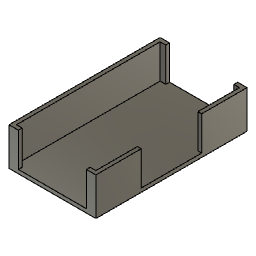
amp box v1 (Autodesk Fusion 360 design; units mm, degrees)
Autodesk Fusion 360 part; units mm, degrees
sketch "Sketch1" plane through (0, 0, 0) normal (0, 0, 1) x (1, 0, 0)
  line L0 (0, 0) -> (46, 0)
  line L1 (46, 0) -> (46, 80)
  line L2 (46, 80) -> (0, 80)
  line L3 (0, 80) -> (0, 0)
  dimension "d1" = 46
  dimension "d2" = 80
  constraint horizontal L0
  constraint vertical L1
  constraint horizontal L2
  constraint vertical L3
  constraint coincident L0.start L3.end
  measures "d1" distance of L0.start L0.end
  measures "d2" distance of L0.start L2.end
extrude "Extrude1" add sketch "Sketch1" along normal blind 20
shell "Shell1" thickness 2 removed faces 1 at (15.3333, 53.3333, 20)
sketch "Sketch2" plane through (0, 0, 0) normal (0, -1, 0) x (1, 0, 0)
  line L0 (0, 0) -> (46, 0)
  line L1 (46, 0) -> (46, 20)
  line L2 (46, 20) -> (0, 20)
  line L3 (0, 20) -> (0, 0)
  line L4 (46, 20) -> (41, 20)
  line L5 (41, 20) -> (41, -16.068)
  line L6 (41, -16.068) -> (46, -16.068)
  line L7 (46, -16.068) -> (46, 20)
  line L8 (0, 0) -> (5, 0)
  line L9 (5, 0) -> (5, 36.068)
  line L10 (5, 36.068) -> (0, 36.068)
  line L11 (0, 36.068) -> (0, 0)
  line L12 (46, 0) -> (0, 0)
  line L13 (0, 0) -> (0, 2)
  line L14 (0, 2) -> (46, 2)
  line L15 (46, 2) -> (46, 0)
  dimension "d6" = 5
  dimension "d7" = 5
  dimension "d8" = 2
  constraint horizontal L4
  constraint vertical L5
  constraint horizontal L6
  constraint vertical L7
  constraint coincident L1.end L2.start
  constraint horizontal L8
  constraint vertical L9
  constraint horizontal L10
  constraint vertical L11
  constraint coincident L0.start L3.end
  constraint horizontal L12
  constraint vertical L13
  constraint horizontal L14
  constraint vertical L15
  constraint coincident L0.end L1.start
  measures "d6" distance of L1.end L4.end
  measures "d7" distance of L0.start L8.end
  measures "d8" distance of L0.end L14.end
extrude "Extrude2" cut sketch "Sketch2" against normal blind 155 contours L2 L5 L9 L14
sketch "Sketch3" plane through (46, 0, 0) normal (1, 0, 0) x (0, 1, 0)
  line L0 (0, 0) -> (80, 0)
  line L1 (80, 0) -> (80, 20)
  line L2 (80, 20) -> (0, 20)
  line L3 (0, 20) -> (0, 0)
  line L4 (80, 0) -> (56, 0)
  line L5 (56, 0) -> (56, 36.068)
  line L6 (56, 36.068) -> (80, 36.068)
  line L7 (80, 36.068) -> (80, 0)
  line L8 (0, 20) -> (24, 20)
  line L9 (24, 20) -> (24, -16.068)
  line L10 (24, -16.068) -> (0, -16.068)
  line L11 (0, -16.068) -> (0, 20)
  line L12 (0, 0) -> (142, 0)
  line L13 (142, 0) -> (142, 2)
  line L14 (142, 2) -> (0, 2)
  line L15 (0, 2) -> (0, 0)
  dimension "d11" = 24
  dimension "d12" = 24
  dimension "d13" = 2
  constraint horizontal L4
  constraint vertical L5
  constraint horizontal L6
  constraint vertical L7
  constraint coincident L0.end L1.start
  constraint horizontal L8
  constraint vertical L9
  constraint horizontal L10
  constraint vertical L11
  constraint coincident L2.end L3.start
  constraint horizontal L12
  constraint vertical L13
  constraint horizontal L14
  constraint vertical L15
  constraint coincident L0.start L3.end
  measures "d11" distance of L0.end L4.end
  measures "d12" distance of L2.end L8.end
  measures "d13" distance of L0.start L14.end
extrude "Extrude3" cut sketch "Sketch3" against normal blind 15 contours L2 L5 L9 L14
